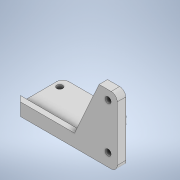
# Autodesk Inventor part: bridge_structure_B
Saved by Autodesk Inventor 2021 (Build 250183000, 183)
## iProperties
Created: 2026-02-14
Part Number: bridge_structure_B
Material: Generic
Document SubType Name: Modeling
Designer: Toby
Density: 1 g/cm^3
Appearance: Default
Author: Toby
Autodesk Inventor part; units mm, degrees
ref_plane "YZ Plane" through (0, 0, 0) normal (1, 0, 0) x (0, 1, 0)
ref_plane "XZ Plane" through (0, 0, 0) normal (0, 1, 0) x (-1, 0, 0)
ref_plane "XY Plane" through (0, 0, 0) normal (0, 0, 1) x (1, 0, 0)
sketch "Sketch1" plane through (0, 0, 0) normal (0, 0, 1) x (1, 0, 0)
  line L0 (22.5, 10) -> (28.5, 10)
  line L1 (28.5, 10) -> (28.5, -10)
  line L2 (28.5, -10) -> (22.5, -10)
  line L3 (22.5, -10) -> (22.5, 10)
  line L4 (22.5, -10) -> (-28.5, -10)
  line L5 (-28.5, -10) -> (-28.5, -8)
  line L6 (-28.5, -8) -> (22.5, -8)
  line L7 (22.5, -8) -> (22.5, -10)
  circle A0 centre (25.5, 7) radius 1
  circle A1 centre (25.5, -8) radius 1
  point P0 (0, 0)
  dimension "d0" = 57
  dimension "d1" = 2
  dimension "d2" = 28.5
  dimension "d3" = 20
  dimension "d4" = 10
  dimension "d5" = 54
  dimension "d6" = 54
  dimension "d7" = 2
  dimension "d8" = 17
  dimension "d9" = 3
  dimension "d10" = 3
  dimension "d11" = 2
  dimension "d12" = 2
  constraints: 16 end point, 4 parallel, 2 centre point, 2 coincident, 2 horizontal, 2 perpendicular
  measures "d0" distance between parallel lines of L1 L5
  measures "d1" distance between parallel lines of L4 L6
  measures "d2" horizontal distance of point (0, 0) L4.end
  measures "d3" distance between parallel lines of L2 L0
  measures "d4" distance from line of L0 point (0, 0)
  measures "d5" horizontal distance of L4.end point (25.5, -8)
  measures "d6" horizontal distance of L4.end point (25.5, 7)
  measures "d7" distance from line of L2 point (25.5, -8)
  measures "d8" distance from line of L2 point (25.5, 7)
  measures "d9" distance from line of L1 point (25.5, 7)
  measures "d10" distance from line of point (25.5, 7) L3
  measures "d11" diameter of A0
  measures "d12" diameter of A1
extrude "Extrusion1" add sketch "Sketch1" along normal blind 3
sketch "Sketch2" plane through (0, 0, 3) normal (0, 0, 1) x (1, 0, 0)
  line L0 (-28.5, -10) -> (28.5, -10) projected
  line L1 (28.5, 10) -> (22.5, 10) projected
  line L2 (13.5, -10) -> (22.5, 10)
  line L3 (22.5, -8) -> (-28.5, -8) projected
  line L4 (22.5, 10) -> (22.5, -8)
  line L5 (22.5, -8) -> (13.5, -10)
  point P0 (0, 0)
  point P1 (14.4, -8)
  dimension "d15" = 42
  constraints: 6 end point, 1 perpendicular, 1 point on line
  measures "d15" distance of L0.start L2.start
extrude "Extrusion2" add sketch "Sketch2" against normal blind 3 contours L2 L4 L3
sketch "Sketch4" plane through (-28.5, -10, 0) normal (0, -1, 0) x (1, 0, 0)
  line L0 (0, 3) -> (57, 3) projected
  line L1 (0, 3) -> (57, 3)
  line L2 (57, 3) -> (57, -13)
  line L3 (57, -13) -> (0, -13)
  line L4 (0, -13) -> (0, 3)
  line L5 (57, 0) -> (57, 3) projected
  point P0 (28.5, 0)
  dimension "d22" = 16
  constraints: 8 end point, 2 parallel, 1 collinear, 1 horizontal, 1 perpendicular
  measures "d22" distance between parallel lines of L3 L0
extrude "Extrusion4" add sketch "Sketch4" along normal blind 2.2
sketch "Sketch5" plane through (-28.5, -10, 0) normal (0, 1, 0) x (1, 0, 0)
  line L0 (0, 0) -> (57, 0) projected
  line L1 (0, 13) -> (57, 13) projected
  line L2 (0, 0) -> (57, 0)
  line L3 (57, 0) -> (57, 13)
  line L4 (57, 13) -> (0, 13)
  line L5 (0, 13) -> (0, 0)
  point P0 (28.5, 0)
  constraints: 8 end point, 2 parallel, 1 horizontal, 1 perpendicular
extrude "Extrusion5" cut sketch "Sketch5" against normal blind 0.2
sketch "Sketch6" plane through (0, 0, 0) normal (0, 0, -1) x (-1, 0, 0)
  line L0 (-28.5, 10) -> (-28.5, -12.2) projected
  line L1 (-28.5, -10.2) -> (28.5, -10.2) projected
  line L2 (-28.5, 10) -> (28.5, 10)
  line L3 (28.5, 10) -> (28.5, -10.2)
  line L4 (28.5, -10.2) -> (-28.5, -10.2)
  line L5 (-28.5, -10.2) -> (-28.5, 10)
  point P0 (0, 0)
  constraints: 8 end point, 2 parallel, 1 horizontal, 1 perpendicular
extrude "Extrusion6" cut sketch "Sketch6" against normal blind 0.2
sketch "Sketch7" plane through (-28.5, -12.2, 0) normal (0, -1, 0) x (1, 0, 0)
  line L0 (0, 3) -> (0, -13) projected
  line L1 (57, 3) -> (0, 3) projected
  point P0 (28.5, 0)
  point P1 (25, 0)
  point P2 (25, -10)
  point P3 (40, 0)
  point P4 (40, -10)
  dimension "d29" = 25
  dimension "d30" = 40
  dimension "d31" = 25
  dimension "d32" = 40
  dimension "d33" = 10
  dimension "d34" = 10
  dimension "d35" = 3
  dimension "d36" = 3
  measures "d29" distance from line of L0 point (25, 0)
  measures "d30" distance from line of L0 point (40, 0)
  measures "d31" distance from line of L0 point (25, -10)
  measures "d32" distance from line of L0 point (40, -10)
  measures "d33" distance of point (25, -10) point (25, 0)
  measures "d34" distance of point (40, -10) point (40, 0)
  measures "d35" distance from line of L1 point (25, 0)
  measures "d36" distance from line of L1 point (40, 0)
hole "Hole1" at (-3.5, -12.2, 0) at (-3.5, -12.2, -10) at (11.5, -12.2, 0) at (11.5, -12.2, -10) direction (0, 1, 0) diameter 2 depth 5 tip angle 118
sketch "Sketch8" plane through (-28.5, -8, 3) normal (0, 1, 0) x (1, 0, 0)
  line L0 (42.9, 2.8) -> (40.9798, 2.8) projected
  line L1 (42.9, 2.8) -> (20.9, 2.8)
  line L2 (20.9, 2.8) -> (20.9, 1.8)
  line L3 (20.9, 1.8) -> (42.9, 1.8)
  line L4 (42.9, 1.8) -> (42.9, 2.8)
  point P0 (28.5, 3)
  dimension "d44" = 22
  dimension "d45" = 1
  constraints: 8 end point, 2 parallel, 1 horizontal, 1 perpendicular
  measures "d44" distance between parallel lines of L4 L2
  measures "d45" distance between parallel lines of L1 L3
extrude "Extrusion7" cut sketch "Sketch8" against normal blind 2.2
chamfer "Chamfer1" distance 1 angle 45 2 edges at (-7.6, -9.1, 0.2) (14.4, -9.1, 1.2)
sketch "Sketch9" plane through (-28.5, -12.2, 0) normal (0, -1, 0) x (1, 0, 0)
  line L0 (0, 3) -> (0, -13) projected
  line L1 (0, -13) -> (57, -13) projected
  line L2 (0, 3) -> (23, 3)
  line L3 (23, 3) -> (23, -13)
  line L4 (23, -13) -> (0, -13)
  line L5 (0, -13) -> (0, 3)
  point P0 (28.5, 0)
  dimension "d51" = 23
  constraints: 8 end point, 2 parallel, 1 horizontal, 1 perpendicular, 1 point on line
  measures "d51" distance between parallel lines of L0 L3
extrude "Extrusion8" cut sketch "Sketch9" against normal blind 5
chamfer "Chamfer2" distance 2 angle 45 1 edges at (-5.5, -10.1, 3)
sketch "Sketch10" plane through (-28.5, -10.2, 0) normal (0, 1, 0) x (1, 0, 0)
  line L0 (57, -0.2) -> (51, -0.2) projected
  line L1 (23, 13) -> (57, 13) projected
  line L2 (57, -0.2) -> (45, -0.2)
  line L3 (45, -0.2) -> (45, 13)
  line L4 (45, 13) -> (57, 13)
  line L5 (57, 13) -> (57, -0.2)
  circle A0 centre (40, 0) radius 1 projected
  point P0 (28.5, 0)
  dimension "d57" = 5
  constraints: 8 end point, 2 parallel, 1 horizontal, 1 perpendicular, 1 point on line
  measures "d57" distance from line of A0.centre L3
extrude "Extrusion9" cut sketch "Sketch10" against normal blind 3 contours L0 L2 L3 L1 L5
chamfer "Chamfer3" distance 12 angle 45 1 edges at (16.5, -11.2, 0.2)
fillet "Fillet2" radius 2 2 edges at (16.5, -11.2, -13) (-5.5, -11.2, -13)
fillet "Fillet3" radius 2 2 edges at (28.5, 10, 1.6) (28.5, -12.2, 1.6)
body "Solid1"
